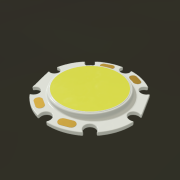
# Autodesk Inventor part: COB LED 3W circular
Saved by Autodesk Inventor 2015 (Build 190159000, 159)
## iProperties
Created: 2015-03-21
Part Number: COB LED 3W circular
Material: Generic
Document SubType Name: Modeling
Designer: Admin
Density: 1 g/cm^3
Appearance: Default
Author: Admin
Autodesk Inventor part; units mm, degrees
ref_plane "YZ Plane" through (0, 0, 0) normal (1, 0, 0) x (0, 1, 0)
ref_plane "XZ Plane" through (0, 0, 0) normal (0, 1, 0) x (-1, 0, 0)
ref_plane "XY Plane" through (0, 0, 0) normal (0, 0, 1) x (1, 0, 0)
sketch "Sketch1" plane through (0, 0, 0) normal (0, 0, 1) x (1, 0, 0)
  arc A0 (-1.1592, 13.9519) -> (1.1592, 13.9519) centre (0, 13) ccw
  arc A1 (-10.6852, 9.0458) -> (-9.0458, 10.6852) centre (-9.1924, 9.1924) ccw
  arc A2 (-13.9519, -1.1592) -> (-13.9519, 1.1592) centre (-13, 0) ccw
  arc A3 (-9.0458, -10.6852) -> (-10.6852, -9.0458) centre (-9.1924, -9.1924) ccw
  arc A4 (1.1592, -13.9519) -> (-1.1592, -13.9519) centre (0, -13) ccw
  arc A5 (10.6852, -9.0458) -> (9.0458, -10.6852) centre (9.1924, -9.1924) ccw
  arc A6 (13.9519, 1.1592) -> (13.9519, -1.1592) centre (13, 0) ccw
  arc A7 (9.0458, 10.6852) -> (10.6852, 9.0458) centre (9.1924, 9.1924) ccw
  arc A8 (-1.1592, 13.9519) -> (-9.0458, 10.6852) centre (0, 0) ccw
  arc A9 (-10.6852, 9.0458) -> (-13.9519, 1.1592) centre (0, 0) ccw
  arc A10 (9.0458, 10.6852) -> (1.1592, 13.9519) centre (0, 0) ccw
  arc A11 (10.6852, -9.0458) -> (13.9519, -1.1592) centre (0, 0) ccw
  arc A12 (-9.0458, -10.6852) -> (-1.1592, -13.9519) centre (0, 0) ccw
  arc A13 (1.1592, -13.9519) -> (9.0458, -10.6852) centre (0, 0) ccw
  line L0 (-13.9519, -1.1592) -> (-10.6852, -9.0458)
  line L1 (13.9519, 1.1592) -> (10.6852, 9.0458)
  dimension "d21" = 360
  constraints: 28 point on circle, 14 centre point, 4 end point, 1 coincident, 33 other
extrude "Extrusion1" add sketch "Sketch1" along normal blind 1
fillet "Fillet1" radius 0.2 48 edges at (9.0458, 10.6852, 0.5) (1.1592, 13.9519, 0.5) (5.3576, 12.9343, 0) (5.3576, 12.9343, 1) (10.6852, 9.0458, 0.5) (8.1317, 8.1317, 0) (8.1317, 8.1317, 1) (13.9519, 1.1592, 0.5) (12.3186, 5.1025, 0) (12.3186, 5.1025, 1) (13.9519, -1.1592, 0.5) (11.5, 0, 0) (11.5, 0, 1) (10.6852, -9.0458, 0.5) (12.9343, -5.3576, 0) (12.9343, -5.3576, 1) (9.0458, -10.6852, 0.5) (8.1317, -8.1317, 0) (8.1317, -8.1317, 1) (1.1592, -13.9519, 0.5) (5.3576, -12.9343, 0) (5.3576, -12.9343, 1) (-1.1592, -13.9519, 0.5) (0, -11.5, 0) (0, -11.5, 1) (-9.0458, -10.6852, 0.5) (-5.3576, -12.9343, 0) (-5.3576, -12.9343, 1) (-10.6852, -9.0458, 0.5) (-8.1317, -8.1317, 0) (-8.1317, -8.1317, 1) (-13.9519, -1.1592, 0.5) (-12.3186, -5.1025, 0) (-12.3186, -5.1025, 1) (-13.9519, 1.1592, 0.5) (-11.5, 0, 0) (-11.5, 0, 1) (-10.6852, 9.0458, 0.5) (-12.9343, 5.3576, 0) (-12.9343, 5.3576, 1) (-9.0458, 10.6852, 0.5) (-8.1317, 8.1317, 0) (-8.1317, 8.1317, 1) (-1.1592, 13.9519, 0.5) (-5.3576, 12.9343, 0) (-5.3576, 12.9343, 1) (0, 11.5, 0) (0, 11.5, 1)
sketch "Sketch2" plane through (0, 0, 1) normal (0, 0, 1) x (1, 0, 0)
  arc A0 (1.543, -13.7135) -> (11.1047, -8.193) centre (0, 0) ccw projected
  circle A1 centre (0, 0) radius 10
  circle A2 centre (0, 0) radius 9.4868
  dimension "d9" = 20
  dimension "d10" = 0.5132
  constraints: 2 centre point, 1 coincident
  measures "d9" diameter of A1
  measures "d10" radial gap between concentric circles of A1 A2
extrude "Extrusion2" add sketch "Sketch2" along normal blind 1.2
sketch "Sketch3" plane through (0, 0, 1) normal (0, 0, 1) x (1, 0, 0)
  circle A0 centre (0, 0) radius 9.4868 projected
extrude "Extrusion3" add sketch "Sketch3" along normal blind 1.3
fillet "Fillet2" radius 0.43 3 edges at (-10, 0, 1) (-10, 0, 2.2) (-9.4868, 0, 2.3)
sketch "Sketch4" plane through (0, 0, 1) normal (0, 0, 1) x (1, 0, 0)
  arc A0 (8.6058, 10.788) -> (1.543, 13.7135) centre (0, 0) ccw projected
  arc A1 (-1.543, 13.7135) -> (1.543, 13.7135) centre (0, 13) ccw projected
  arc A2 (8.6058, 10.788) -> (10.7184, 8.4431) centre (9.1924, 9.1924) ccw projected
  circle A3 centre (0, 0) radius 10.43 projected
  line L0 (3.7506, 11.6097) -> (5.5267, 10.7932)
  line L1 (3.7506, 11.6097) -> (5.5267, 10.7932) construction
  line L2 (3.3171, 10.6667) -> (5.0931, 9.8502)
  line L3 (5.9602, 11.7362) -> (4.1841, 12.5527)
  arc A4 (4.1841, 12.5527) -> (3.3171, 10.6667) centre (3.7506, 11.6097) ccw
  arc A5 (5.0931, 9.8502) -> (5.9602, 11.7362) centre (5.5267, 10.7932) ccw
  point P0 (4.6386, 11.2014)
  dimension "d23" = 1.685
  dimension "d24" = 1.685
  dimension "d25" = 4
  dimension "d26" = 4
  constraints: 10 end point, 4 point on circle, 4 tangent, 2 centre point, 2 equal length, 1 midpoint
  measures "d23" distance edge to line of A3 L0
  measures "d24" distance edge to line of A0 L0
  measures "d25" distance of A1.centre L0.start
  measures "d26" distance of A2.centre L0.end
extrude "Extrusion4" add sketch "Sketch4" along normal blind 0.05 contours A4 L3 A5 L2
mirror "Mirror1" about plane through (0, 0, 0) normal (1, 0, 0) of "Extrusion4"
mirror "Mirror2" about plane through (0, 0, 0) normal (0, 1, 0) of "Extrusion4", "Mirror1"
equation "\"d23\" = d24"
equation "\"d26\" = d25"
body "Solid1"
